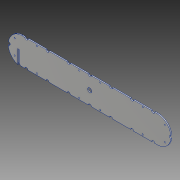
# Autodesk Inventor part: 1312_Former Middle_V1
Saved by Autodesk Inventor 2020 (Build 240168000, 168)
## iProperties
Created: 2019-09-10
Part Number: 1312_Former Middle_V1
Material: Aluminum 6061
Document SubType Name: Modeling
Designer: MPI
Density: 2.7 g/cm^3
Appearance: Aluminum - Flat
Mass: 5622.53 g
Surface Area: 6914.04 cm^2
Volume: 5622.53 cm^3
Author: MPI
Autodesk Inventor part; units mm, degrees
ref_plane "YZ Plane" through (0, 0, 0) normal (1, 0, 0) x (0, 1, 0)
ref_plane "XZ Plane" through (0, 0, 0) normal (0, 1, 0) x (-1, 0, 0)
ref_plane "XY Plane" through (0, 0, 0) normal (0, 0, 1) x (1, 0, 0)
sketch "Sketch1" plane through (0, 0, 0) normal (0, 1, 0) x (-1, 0, 0)
  line L0 (432, 86) -> (-432, 86)
  line L1 (-432, -86) -> (432, -86)
  arc A0 (432, -86) -> (432, 86) centre (432, 0) ccw
  arc A1 (-432, 86) -> (-432, -86) centre (-432, 0) ccw
  point P0 (0, 0)
  dimension "d4" = 432
  dimension "d5" = 864
  dimension "d7" = 86
  dimension "d107" = 172
  constraints: 4 end point, 4 point on circle, 3 tangent, 2 centre point, 1 horizontal, 1 parallel
  measures "d4" distance of point (0, 0) A0.centre
  measures "d5" distance of A1.centre A0.centre
  measures "d7" radius of A0
  measures "d107" distance between parallel lines of L0 L1
extrude "Extrusion1" add sketch "Sketch1" along normal blind 6.2
sketch "Sketch4" plane through (0, 6.2, 0) normal (0, 1, 0) x (1, 0, 0)
  line L0 (-659.0781, -10) -> (-659.0781, 10)
  line L1 (670.9769, 10) -> (670.9769, -10)
  line L2 (-10, 220.6364) -> (10, 220.6364)
  line L3 (-125, -216.3636) -> (-145, -216.3636)
  line L4 (-145, 220.6364) -> (-125, 220.6364)
  line L5 (-260, -216.3636) -> (-280, -216.3636)
  line L6 (-280, 220.6364) -> (-260, 220.6364)
  line L7 (145, -216.3636) -> (125, -216.3636)
  line L8 (125, 220.6364) -> (145, 220.6364)
  line L9 (280, -216.3636) -> (260, -216.3636)
  line L10 (260, 220.6364) -> (280, 220.6364)
  line L11 (395, 220.6364) -> (415, 220.6364)
  line L12 (-432, -86) -> (432, -86) projected
  line L13 (432, 86) -> (-432, 86) projected
  line L14 (395, 86) -> (395, 220.6364)
  line L15 (415, 220.6364) -> (415, 86)
  line L16 (280, -86) -> (280, -216.3636)
  line L17 (260, -216.3636) -> (260, -86)
  line L18 (280, 220.6364) -> (280, 86)
  line L19 (260, 86) -> (260, 220.6364)
  line L20 (145, -86) -> (145, -216.3636)
  line L21 (125, -216.3636) -> (125, -86)
  line L22 (145, 220.6364) -> (145, 86)
  line L23 (125, 86) -> (125, 220.6364)
  line L24 (10, 220.6364) -> (10, 86)
  line L25 (-10, 86) -> (-10, 220.6364)
  line L26 (-125, -86) -> (-125, -216.3636)
  line L27 (-145, -216.3636) -> (-145, -86)
  line L28 (-125, 220.6364) -> (-125, 86)
  line L29 (-145, 86) -> (-145, 220.6364)
  line L30 (-260, -86) -> (-260, -216.3636)
  line L31 (-280, -216.3636) -> (-280, -86)
  line L32 (-260, 220.6364) -> (-260, 86)
  line L33 (-280, 86) -> (-280, 220.6364)
  arc A0 (395, 86) -> (415, 86) centre (405, 86) ccw
  arc A1 (260, 86) -> (280, 86) centre (270, 86) ccw
  arc A2 (125, 86) -> (145, 86) centre (135, 86) ccw
  arc A3 (-10, 86) -> (10, 86) centre (0, 86) ccw
  arc A4 (-145, 86) -> (-125, 86) centre (-135, 86) ccw
  arc A5 (-280, 86) -> (-260, 86) centre (-270, 86) ccw
  arc A6 (-260, -86) -> (-280, -86) centre (-270, -86) ccw
  arc A7 (-125, -86) -> (-145, -86) centre (-135, -86) ccw
  arc A8 (145, -86) -> (125, -86) centre (135, -86) ccw
  arc A9 (280, -86) -> (260, -86) centre (270, -86) ccw
  arc A10 (518, 10) -> (518, -10) centre (518, 0) ccw
  arc A11 (-518, -10) -> (-518, 10) centre (-518, 0) ccw
  line L34 (-659.0781, 10) -> (-518, 10)
  line L35 (517.4166, 10) -> (670.9769, 10)
  line L36 (670.9769, -10) -> (518, -10)
  line L37 (-518, -10) -> (-659.0781, -10)
  circle A12 centre (-480, 48) radius 4
  circle A13 centre (-337.5, 76) radius 4
  circle A14 centre (337.5, 76) radius 4
  circle A15 centre (480, 48) radius 4
  circle A16 centre (480, -48) radius 4
  circle A17 centre (337.5, -76) radius 4
  circle A18 centre (-337.5, -76) radius 4
  circle A19 centre (-480, -48) radius 4
  arc A20 (-432, 86) -> (-432, -86) centre (-432, 0) ccw projected
  line L38 (10, -86) -> (10, -216.3636)
  line L39 (-10, -216.3636) -> (-10, -86)
  arc A21 (10, -86) -> (-10, -86) centre (0, -86) ccw
  line L40 (-10, -216.3636) -> (10, -216.3636)
  line L41 (-415, 220.6364) -> (-395, 220.6364)
  line L42 (-395, 220.6364) -> (-395, 86)
  line L43 (-415, 86) -> (-415, 220.6364)
  arc A22 (-415, 86) -> (-395, 86) centre (-405, 86) ccw
  line L44 (415, -216.3636) -> (395, -216.3636)
  line L45 (415, -86) -> (415, -216.3636)
  line L46 (395, -216.3636) -> (395, -86)
  arc A23 (415, -86) -> (395, -86) centre (405, -86) ccw
  line L47 (-395, -216.3636) -> (-415, -216.3636)
  line L48 (-395, -86) -> (-395, -216.3636)
  line L49 (-415, -216.3636) -> (-415, -86)
  arc A24 (-395, -86) -> (-415, -86) centre (-405, -86) ccw
  line L50 (-432, 0) -> (-518, 0)
  circle A25 centre (-67.5, 76) radius 4
  circle A26 centre (67.5, 76) radius 4
  circle A27 centre (67.5, -76) radius 4
  circle A28 centre (-67.5, -76) radius 4
  point P0 (480, -91)
  point P1 (480, 91)
  point P2 (-395, 86)
  point P3 (-395, 86)
  dimension "d18" = 20
  dimension "d54" = 76
  dimension "d55" = 48
  dimension "d59" = 48
  dimension "d60" = 76
  dimension "d73" = 8
  dimension "d109" = 135
  dimension "d110" = 135
  dimension "d111" = 135
  dimension "d112" = 135
  dimension "d113" = 135
  dimension "d115" = 135
  dimension "d116" = 20
  dimension "d120" = 48
  dimension "d121" = 38
  dimension "d122" = 38
  dimension "d123" = 48
  dimension "d124" = 38
  dimension "d125" = 38
  dimension "d130" = 76
  dimension "d131" = 76
  dimension "d144" = 76
  dimension "d145" = 76
  dimension "d146" = 76
  dimension "d147" = 76
  dimension "d149" = 57.5
  dimension "d150" = 57.5
  dimension "d151" = 57.5
  dimension "d152" = 57.5
  dimension "d153" = 57.5
  dimension "d154" = 57.5
  dimension "d155" = 57.5
  dimension "d156" = 57.5
  constraints: 98 end point, 33 point on circle, 31 parallel, 28 centre point, 25 collinear, 24 tangent, 12 perpendicular, 11 equal radius, 10 horizontal, 3 point on line, 2 vertical, 23 other
  measures "d18" distance of L0.start L0.end
  measures "d54" vertical distance of A14.centre A10.centre
  measures "d55" vertical distance of A10.centre A15.centre
  measures "d59" vertical distance of A16.centre A10.centre
  measures "d60" vertical distance of A17.centre A10.centre
  measures "d73" diameter of A12
  measures "d109" distance between parallel lines of L22 L24
  measures "d110" distance between parallel lines of L18 L22
  measures "d111" distance between parallel lines of L15 L18
  measures "d112" distance between parallel lines of L29 L25
  measures "d113" distance between parallel lines of L33 L29
  measures "d115" distance between parallel lines of L43 L33
  measures "d116" distance of L2.start L2.end
  measures "d120" vertical distance of A19.centre L50.end
  measures "d121" horizontal distance of A19.centre L50.end
  measures "d122" horizontal distance of A12.centre L50.end
  measures "d123" vertical distance of L50.end A12.centre
  measures "d124" horizontal distance of A10.centre A15.centre
  measures "d125" horizontal distance of A10.centre A16.centre
  measures "d130" vertical distance of L50.end A13.centre
  measures "d131" distance from line of L50 A18.centre
  measures "d144" vertical distance of A10.centre A26.centre
  measures "d145" vertical distance of A10.centre A27.centre
  measures "d146" vertical distance of L50.end A25.centre
  measures "d147" vertical distance of L50.end A28.centre
  measures "d149" distance from line of A13.centre L33
  measures "d150" distance from line of L31 A18.centre
  measures "d151" distance from line of A25.centre L28
  measures "d152" distance from line of A28.centre L26
  measures "d153" distance from line of A26.centre L23
  measures "d154" distance from line of A27.centre L21
  measures "d155" distance from line of A14.centre L18
  measures "d156" distance from line of L16 A17.centre
extrude "Extrusion3" cut sketch "Sketch4" against normal through all
sketch "Sketch10" plane through (0, 6.2, 0) normal (0, 1, 0) x (1, 0, 0)
  circle A0 centre (0, 0) radius 13
  constraints: 1 centre point, 1 coincident
extrude "Extrusion7" cut sketch "Sketch10" against normal through all
sketch "Sketch13" plane through (0, 6.2, 0) normal (0, 1, 0) x (1, 0, 0)
  line L0 (-460, 0) -> (-451, 0)
  arc A0 (-432, 86) -> (-517.4186, 9.9831) centre (-432, 0) ccw projected
  arc A1 (-436.8451, 85.8634) -> (-451, 70.8872) centre (-436, 70.8872) ccw
  line L1 (-460, 76.909) -> (-460, 0)
  line L2 (-451, 0) -> (-451, 70.8872)
  arc A2 (-451, 90.6568) -> (-460, 76.909) centre (-445, 76.909) ccw
  arc A3 (-517.4186, -9.9831) -> (-432, -86) centre (-432, 0) ccw projected
  line L3 (-436.8451, 85.8634) -> (-436.8451, 93.1)
  line L4 (-451, 90.6568) -> (-436.8451, 93.1)
  point P0 (0, 0)
  dimension "d163" = 9
  dimension "d167" = 30
  dimension "d168" = 460
  dimension "d169" = 15
  dimension "d175" = 0
  constraints: 10 end point, 5 point on circle, 2 centre point, 2 tangent, 1 horizontal, 1 parallel, 1 perpendicular, 1 vertical
  measures "d163" distance of L0.start L0.end
  measures "d167" diameter of A1
  measures "d168" distance from line of point (0, 0) L1
  measures "d169" radius of A2
  measures "d175" distance from line of A0.centre L0
extrude "Extrusion10" cut sketch "Sketch13" against normal through all
sketch "Sketch14" plane through (0, 6.2, 0) normal (0, 1, 0) x (1, 0, 0)
  line L0 (-451, 0) -> (-460, 0) projected
  line L1 (-460, 0) -> (-515.1777, -9.5935) construction
  line L2 (-460, 0) -> (-460, 76.909) projected
  line L3 (-460, 0) -> (-486.8762, 73.8417)
  arc A0 (-459.2589, 81.5656) -> (-517.4186, 9.9831) centre (-432, 0) ccw projected
  arc A1 (-517.4186, -9.9831) -> (-432, -86) centre (-432, 0) ccw projected
  line L4 (-280, 86) -> (-395, 86) projected
  line L5 (-395, -86) -> (-280, -86) projected
  line L6 (-460, 0) -> (-507.9899, -40.2683)
  line L7 (-460, 0) -> (-536.3277, 0) construction
  line L8 (-459.2589, 81.5656) -> (-459.2589, 87.869)
  arc A2 (-460, 87.6356) -> (-486.8762, 73.8417) centre (-434.6538, 5.1707) ccw
  line L9 (-517.4186, -9.9831) -> (-519.5785, -9.9831)
  line L10 (-517.4186, 9.9831) -> (-520.7839, 9.9831)
  arc A3 (-519.6047, -9.8704) -> (-519.5983, -9.8714) centre (-518, 0) ccw
  arc A4 (-459.2589, 87.869) -> (-520.7839, 9.9831) centre (-434.6234, 5.1651) ccw
  arc A5 (-519.5983, -9.8714) -> (-507.9899, -40.2683) centre (-434.6234, 5.1651) ccw
  arc A6 (-517.4186, -9.9831) -> (-507.9899, -40.2683) centre (-432, 0) ccw
  arc A7 (-459.2589, 81.5656) -> (-517.4186, 9.9831) centre (-432, 0) ccw
  point P0 (0, 0)
  point P1 (-484.7279, 67.9394)
  dimension "d182" = 40
  dimension "d183" = 70
  constraints: 14 end point, 14 point on circle, 6 centre point, 3 horizontal, 2 coincident, 2 point on line, 1 vertical
  measures "d182" angle of L6 L7
  measures "d183" angle of L3 L7
extrude "Extrusion11" add sketch "Sketch14" against normal up to surface (6.2 mm away)
body "Solid1"
